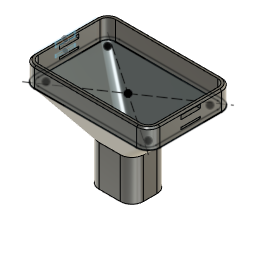
ComponentFunnel (Autodesk Fusion 360 design; units mm, degrees)
Autodesk Fusion 360 part; units mm, degrees
sketch "Sketch1" plane through (0, 0, 0) normal (0, 0, 1) x (1, 0, 0)
  line L0 (5.5, -9.5) -> (-5.5, -9.5)
  line L1 (-11.5, -3.5) -> (-11.5, 3.5)
  line L2 (-5.5, 9.5) -> (5.5, 9.5)
  line L3 (11.5, 3.5) -> (11.5, -3.5)
  line L4 (11.5, -9.5) -> (-11.5, 9.5) construction
  line L5 (-11.5, -9.5) -> (11.5, 9.5) construction
  arc A0 (-5.5, 9.5) -> (-11.5, 3.5) centre (-5.5, 3.5) ccw
  arc A1 (-11.5, -3.5) -> (-5.5, -9.5) centre (-5.5, -3.5) ccw
  arc A2 (5.5, -9.5) -> (11.5, -3.5) centre (5.5, -3.5) ccw
  arc A3 (11.5, 3.5) -> (5.5, 9.5) centre (5.5, 3.5) ccw
  line L6 (5.5, -8.3) -> (-5.5, -8.3)
  arc A4 (-10.3, -3.5) -> (-5.5, -8.3) centre (-5.5, -3.5) ccw
  line L7 (-10.3, -3.5) -> (-10.3, 3.5)
  arc A5 (-5.5, 8.3) -> (-10.3, 3.5) centre (-5.5, 3.5) ccw
  line L8 (-5.5, 8.3) -> (5.5, 8.3)
  arc A6 (10.3, 3.5) -> (5.5, 8.3) centre (5.5, 3.5) ccw
  line L9 (10.3, 3.5) -> (10.3, -3.5)
  arc A7 (5.5, -8.3) -> (10.3, -3.5) centre (5.5, -3.5) ccw
  dimension "d1" = 19
  dimension "d2" = 23
  dimension "d12" = 1.2
  dimension "d13" = 6
  constraint perpendicular L0 L1
  constraint parallel L0 L2
  constraint parallel L1 L3
  constraint horizontal L0
  constraint coincident L4 origin
  constraint coincident L5 origin
  constraint coincident L4.end L2
  constraint coincident L4.end L1
  constraint tangent L2 A0
  constraint tangent L1 A0
  constraint coincident L5.start L1
  constraint coincident L5.start L0
  constraint tangent L1 A1
  constraint tangent L0 A1
  constraint equal A0 A1
  constraint coincident L4.start L0
  constraint coincident L4.start L3
  constraint tangent L0 A2
  constraint tangent L3 A2
  constraint equal A0 A2
  constraint coincident L5.end L3
  constraint coincident L5.end L2
  constraint tangent L3 A3
  constraint tangent L2 A3
  constraint equal A0 A3
  measures "d1" distance of L5.start L4.end
  measures "d2" distance of L4.end L5.end
  measures "d7" distance of L4.start
  measures "d8" radius of L4.start
  measures "d13" radius of A0
extrude "Extrude1" add sketch "Sketch1" along normal blind 21 makes body 1
ref_plane "WorkPlane1" through (0, 0, 41) normal (0, 0, 1) x (1, 0, 0)
sketch "Sketch2" plane through (0, 0, 41) normal (0, 0, 1) x (1, 0, 0)
  line L0 (26.5, -22) -> (-26.5, -22)
  line L1 (-32.5, -16) -> (-32.5, 16)
  line L2 (-26.5, 22) -> (26.5, 22)
  line L3 (32.5, 16) -> (32.5, -16)
  line L4 (32.5, -22) -> (-32.5, 22) construction
  line L5 (-32.5, -22) -> (32.5, 22) construction
  arc A0 (-32.5, -16) -> (-26.5, -22) centre (-26.5, -16) ccw
  arc A1 (-26.5, 22) -> (-32.5, 16) centre (-26.5, 16) ccw
  arc A2 (32.5, 16) -> (26.5, 22) centre (26.5, 16) ccw
  arc A3 (26.5, -22) -> (32.5, -16) centre (26.5, -16) ccw
  arc A4 (30.5, 16) -> (26.5, 20) centre (26.5, 16) ccw
  line L6 (-26.5, 20) -> (26.5, 20)
  arc A5 (-26.5, 20) -> (-30.5, 16) centre (-26.5, 16) ccw
  line L7 (-30.5, -16) -> (-30.5, 16)
  arc A6 (-30.5, -16) -> (-26.5, -20) centre (-26.5, -16) ccw
  line L8 (26.5, -20) -> (-26.5, -20)
  arc A7 (26.5, -20) -> (30.5, -16) centre (26.5, -16) ccw
  line L9 (30.5, 16) -> (30.5, -16)
  dimension "d6" = 65
  dimension "d7" = 44
  dimension "d8" = 6
  dimension "d17" = 2
  constraint perpendicular L0 L1
  constraint parallel L0 L2
  constraint parallel L1 L3
  constraint horizontal L0
  constraint coincident L4 origin
  constraint coincident L5 origin
  constraint coincident L5.start L0
  constraint coincident L5.start L1
  constraint tangent L0 A0
  constraint tangent L1 A0
  constraint coincident L4.end L1
  constraint coincident L4.end L2
  constraint tangent L1 A1
  constraint tangent L2 A1
  constraint equal A0 A1
  constraint coincident L5.end L2
  constraint coincident L5.end L3
  constraint tangent L2 A2
  constraint tangent L3 A2
  constraint equal A0 A2
  constraint coincident L4.start L3
  constraint coincident L4.start L0
  constraint tangent L3 A3
  constraint tangent L0 A3
  constraint equal A0 A3
  measures "d6" distance of L4.end L5.end
  measures "d7" distance of L5.start L4.end
  measures "d8" radius of A0
extrude "Extrude3" add sketch "Sketch2" along normal blind 10 separate body makes body 2
extrude "Extrude2" add sketch "Sketch2" along normal blind 10 separate body contours L0 L1 L2 L3 A0 A1 A2 A3 | A4 L6 A5 L7 A6 L8 A7 L9 makes body 3
sketch "Sketch3" plane through (0, 0, 21) normal (0, 0, 1) x (-1, 0, 0)
  arc A0 (10.3, 3.5) -> (5.5, 8.3) centre (5.5, 3.5) ccw
  line L0 (10.3, 3.5) -> (10.3, -3.5)
  arc A1 (5.5, -8.3) -> (10.3, -3.5) centre (5.5, -3.5) ccw
  line L1 (5.5, -8.3) -> (-5.5, -8.3)
  arc A2 (-10.3, -3.5) -> (-5.5, -8.3) centre (-5.5, -3.5) ccw
  line L2 (-10.3, -3.5) -> (-10.3, 3.5)
  arc A3 (-5.5, 8.3) -> (-10.3, 3.5) centre (-5.5, 3.5) ccw
  line L3 (-5.5, 8.3) -> (5.5, 8.3)
  arc A4 (-5.5, 9.5) -> (-11.5, 3.5) centre (-5.5, 3.5) ccw
  line L4 (-11.5, 3.5) -> (-11.5, -3.5)
  arc A5 (-11.5, -3.5) -> (-5.5, -9.5) centre (-5.5, -3.5) ccw
  line L5 (-5.5, -9.5) -> (5.5, -9.5)
  arc A6 (5.5, -9.5) -> (11.5, -3.5) centre (5.5, -3.5) ccw
  line L6 (11.5, -3.5) -> (11.5, 3.5)
  arc A7 (11.5, 3.5) -> (5.5, 9.5) centre (5.5, 3.5) ccw
  line L7 (5.5, 9.5) -> (-5.5, 9.5)
  line L8 (11.5, -3.5) -> (11.5, 3.5)
  arc A8 (5.5, -9.5) -> (11.5, -3.5) centre (5.5, -3.5) ccw
  line L9 (-5.5, -9.5) -> (5.5, -9.5)
  arc A9 (-11.5, -3.5) -> (-5.5, -9.5) centre (-5.5, -3.5) ccw
  line L10 (-11.5, 3.5) -> (-11.5, -3.5)
  arc A10 (-5.5, 9.5) -> (-11.5, 3.5) centre (-5.5, 3.5) ccw
  line L11 (5.5, 9.5) -> (-5.5, 9.5)
  arc A11 (11.5, 3.5) -> (5.5, 9.5) centre (5.5, 3.5) ccw
loft "Loft2" add profiles "Sketch3", "Sketch2" section 1 contours A0 L0 A1 L1 A2 L2 A3 L3 | A4 L4 A5 L5 A6 L6 A7 L7 L8 A8 L9 A9 L10 A10 L11 A11 section 2 contours L0 L1 L2 L3 A0 A1 A2 A3 | A4 L6 A5 L7 A6 L8 A7 L9 bodies 1
loft "Loft3" cut profiles "Sketch2" section 1 face at (-1.8333, -2.7667, 21) section 2 contours A4 L6 A5 L7 A6 L8 A7 L9 on bodies 1 bodies 1
sketch "Sketch4" plane through (-32.5, 0, 0) normal (-1, 0, 0) x (0, -1, 0)
  line L0 (-16, 41) -> (16, 41)
  line L1 (16, 41) -> (16, 51)
  line L2 (16, 51) -> (-16, 51)
  line L3 (-16, 51) -> (-16, 41)
  line L4 (5, 48) -> (-5, 48)
  line L5 (-5, 48) -> (-5, 50)
  line L6 (-5, 50) -> (5, 50)
  line L7 (5, 50) -> (5, 48)
  line L8 (5, 48) -> (-5, 50) construction
  line L9 (-5, 48) -> (5, 50) construction
  line L10 (5, 43.5) -> (-5, 43.5)
  line L11 (-5, 43.5) -> (-5, 44.5)
  line L12 (-5, 44.5) -> (5, 44.5)
  line L13 (5, 44.5) -> (5, 43.5)
  line L14 (5, 43.5) -> (-5, 44.5) construction
  line L15 (-5, 43.5) -> (5, 44.5) construction
  point P0 (0, 49)
  point P1 (0, 44)
  dimension "d20" = 10
  dimension "d21" = 1
  dimension "d22" = 10
  constraint perpendicular L4 L5
  constraint parallel L4 L6
  constraint parallel L5 L7
  constraint horizontal L4
  constraint coincident L8 P0
  constraint coincident L9 P0
  constraint perpendicular L10 L11
  constraint parallel L10 L12
  constraint parallel L11 L13
  constraint horizontal L10
  constraint coincident L14 P1
  constraint coincident L15 P1
  measures "d20" distance of L5.end L6.end
  measures "d21" distance of L10.end L11.end
  measures "d22" distance of L11.end L12.end
extrude "Extrude5" cut sketch "Sketch4" against normal up to surface (65 mm away) contours L4 L5 L6 L7 bodies 2
extrude "Extrude4" cut sketch "Sketch4" against normal up to surface (65 mm away) contours L10 L11 L12 L13 bodies 2
chamfer "Chamfer1" distance 0.8 angle 45 8 edges at (-32.5, 0, 51) (-30.7426, -20.2426, 51) (0, -22, 51) (30.7426, -20.2426, 51) (32.5, 0, 51) (30.7426, 20.2426, 51) (0, 22, 51) (-30.7426, 20.2426, 51) on bodies 2
hidden bodies 3
